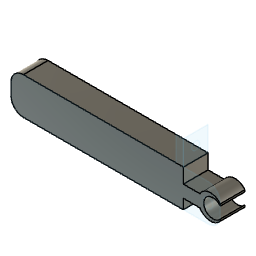
Current Final Hand Assembly (Autodesk Fusion 360 archive; units mm, degrees)
design "index_finger_new v3 (1) v2"
Autodesk Fusion 360 part; units mm, degrees
note: some values were not read from the file. Chosen so that the rebuilt part matches the saved one: where a step ends; which bodies a step acts on; which face or edge a step refers to. Set by a fixed rule: which sketch regions a step uses.
(part 1 of 5)
sketch "Sketch1" plane through (0, 0, 0) normal (0, 1, 0) x (1, 0, 0)
  line L0 (0, 0) -> (85, 0)
  line L1 (85, 0) -> (85, -15)
  line L2 (85, -15) -> (0, -15)
  line L3 (0, -15) -> (0, 0)
  dimension "d1" = 85
  dimension "d2" = 15
  constraint horizontal L0
  constraint vertical L1
  constraint horizontal L2
  constraint vertical L3
  constraint coincident L0.start L3.end
  measures "d1" distance of L0.start L0.end
  measures "d2" distance of L0.start L2.end
extrude "Extrude1" add sketch "Sketch1" along normal blind 10 makes body 1
fillet "Fillet1" radius 5 4 edges at (0, 5, 15) (0, 5, 0) (85, 5, 15) (85, 5, 0) on bodies 1
sketch "Sketch2" plane through (0, 0, 15) normal (0, 0, 1) x (-1, 0, 0)
  line L0 (-80, 0) -> (-80, -10)
  line L1 (-80, -10) -> (-5, -10)
  line L2 (-5, -10) -> (-5, 0)
  line L3 (-5, 0) -> (-80, 0)
  line L4 (-67, -10) -> (-70, -10)
  line L5 (-70, -10) -> (-70, 0)
  line L6 (-70, 0) -> (-67, 0)
  line L7 (-67, 0) -> (-67, -10)
  dimension "d7" = 3
  dimension "d8" = 10
  constraint horizontal L4
  constraint vertical L5
  constraint horizontal L6
  constraint vertical L7
  constraint coincident L1 L4.start
  measures "d7" distance of L4.start L4.end
  measures "d8" distance of L0 L5
extrude "Extrude2" add sketch "Sketch2" along normal blind 10 contours L1 L3 L4 L5 L6 L7 bodies 1
sketch "Sketch3" plane through (0, 0, 0) normal (0, -1, 0) x (1, 0, 0)
  arc A0 (80, 0) -> (85, 5) centre (80, 5) ccw
  line L0 (85, 5) -> (85, 10)
  arc A1 (85, 10) -> (80, 15) centre (80, 10) ccw
  line L1 (80, 15) -> (70, 15)
  line L2 (70, 15) -> (70, 25)
  line L3 (70, 25) -> (67, 25)
  line L4 (67, 25) -> (67, 15)
  line L5 (67, 15) -> (5, 15)
  arc A2 (5, 15) -> (0, 10) centre (5, 10) ccw
  line L6 (0, 10) -> (0, 5)
  arc A3 (0, 5) -> (5, 0) centre (5, 5) ccw
  line L7 (5, 0) -> (80, 0)
  circle A4 centre (80, 7.4726) radius 2
  dimension "d11" = 4
  measures "d11" diameter of A4
extrude "Extrude3" cut sketch "Sketch3" against normal blind 13 contours A4 bodies 1
sketch "Sketch4" plane through (70, 0, 0) normal (1, 0, 0) x (0, 1, 0)
  line L0 (0, 15) -> (10, 15)
  line L1 (10, 15) -> (10, 25)
  line L2 (10, 25) -> (0, 25)
  line L3 (0, 25) -> (0, 15)
  circle A0 centre (5, 20.0248) radius 1.625
  dimension "d14" = 3.25
  measures "d14" diameter of A0
extrude "Extrude4" cut sketch "Sketch4" against normal blind 56 contours A0 bodies 1
sketch "Sketch5" plane through (0, 0, 0) normal (0, -1, 0) x (1, 0, 0)
  circle A0 centre (80, 7.4726) radius 2
  arc A1 (80, 0) -> (85, 5) centre (80, 5) ccw
  line L0 (85, 5) -> (85, 10)
  arc A2 (85, 10) -> (80, 15) centre (80, 10) ccw
  line L1 (80, 15) -> (70, 15)
  line L2 (70, 15) -> (70, 25)
  line L3 (70, 25) -> (67, 25)
  line L4 (67, 25) -> (67, 15)
  line L5 (67, 15) -> (5, 15)
  arc A3 (5, 15) -> (0, 10) centre (5, 10) ccw
  line L6 (0, 10) -> (0, 5)
  arc A4 (0, 5) -> (5, 0) centre (5, 5) ccw
  line L7 (5, 0) -> (80, 0)
sketch "Sketch6" plane through (70, 0, 0) normal (1, 0, 0) x (0, 1, 0)
  circle A0 centre (5, 20.0248) radius 1.625
  line L0 (0, 15) -> (10, 15)
  line L1 (10, 15) -> (10, 25)
  line L2 (10, 25) -> (0, 25)
  line L3 (0, 25) -> (0, 15)
sketch "Sketch7" plane through (85, 0, 0) normal (1, 0, 0) x (0, 1, 0)
  line L0 (0, 5) -> (10, 5)
  line L1 (10, 5) -> (10, 10)
  line L2 (10, 10) -> (0, 10)
  line L3 (0, 10) -> (0, 5)
  line L4 (0, 15) -> (10, 15)
  line L5 (10, 15) -> (10, 0)
  line L6 (10, 0) -> (0, 0)
  line L7 (0, 0) -> (0, 15)
  constraint horizontal L4
  constraint vertical L5
  constraint horizontal L6
  constraint vertical L7
extrude "Extrude5" cut sketch "Sketch7" against normal blind 15 bodies 1
sketch "Sketch8" plane through (70, 0, 0) normal (1, 0, 0) x (0, 1, 0)
  circle A0 centre (5, 20.0248) radius 1.625
  line L0 (10, 0) -> (10, 25)
  line L1 (10, 25) -> (0, 25)
  line L2 (0, 25) -> (0, 0)
  line L3 (0, 0) -> (10, 0)
  line L4 (0, 9) -> (10, 9)
  line L5 (10, 9) -> (10, 4)
  line L6 (10, 4) -> (0, 4)
  line L7 (0, 4) -> (0, 9)
  line L8 (10, 25) -> (0, 25)
  dimension "d19" = 5
  dimension "d20" = 10
  dimension "d21" = 16
  constraint horizontal L4
  constraint vertical L5
  constraint horizontal L6
  constraint vertical L7
  constraint coincident L2 L4.start
  measures "d19" distance of L4.start L6.end
  measures "d20" distance of L4.start L4.end
  measures "d21" distance of L4 L8
extrude "Extrude6" add sketch "Sketch8" along normal blind 7.5 contours L0 L2 L4 L5 L6 L7 bodies 1
cylinder "CylinderPrimitive1" add diameter 10 height -10 placed x (1, 0, 0) y (0, 0, -1) z (0, 1, 0) at (81.0326, 10, 6.5) separate body makes body 2
ref_plane "WorkPlane1" through (87, 0, 0) normal (1, 0, 0) x (0, 1, 0)
sketch "Sketch11" plane through (87, 0, 0) normal (1, 0, 0) x (0, 1, 0)
  line L0 (-1.0999, 12.5133) -> (11, 12.5133)
  line L1 (11, 12.5133) -> (11, 1)
  line L2 (11, 1) -> (-1.0999, 1)
  line L3 (-1.0999, 1) -> (-1.0999, 12.5133)
  constraint horizontal L0
  constraint vertical L1
  constraint horizontal L2
  constraint vertical L3
extrude "Extrude7" cut sketch "Sketch11" against normal blind 2 bodies 2
copy_body "CopyPasteBodies1" bodies 2 makes body 3
move_body "Move1" bodies 3 to x (1, 0, 0) y (0, 1, 0) z (0, 0, 1) at (19, 0, 0)
scale "Scale1" factors (0.75, 1, 0.75) about (104, 0, 3.457) bodies 3
move_body "Move2" bodies 3 to x (1, 0, 0) y (0, 1, 0) z (0, 0, 1) at (-19, 0, 0.7608)
combine "Combine1" operation add target body 1 tool bodies 2
split "Split1" by bodies 3 bodies 1 makes body 4 at (47.3333, 10, 5)
move_body "Move3" bodies 1 to x (1, 0, 0) y (0, 1, 0) z (0, 0, 1) at (20, 0, 0)
sketch "Sketch12" plane through (0, 0, 0) normal (0, -1, 0) x (1, 0, 0)
sketch "Sketch15" plane through (67, 0, 0) normal (-1, 0, 0) x (0, -1, 0)
  circle A0 centre (-5, 20.0248) radius 1.625
  line L0 (-10, 15) -> (0, 15)
  line L1 (0, 15) -> (0, 25)
  line L2 (0, 25) -> (-10, 25)
  line L3 (-10, 25) -> (-10, 15)
  line L4 (-10, 25) -> (0, 25)
  line L5 (0, 25) -> (0, 15)
  line L6 (0, 15) -> (-10, 15)
  line L7 (-10, 15) -> (-10, 25)
  constraint horizontal L4
  constraint vertical L5
  constraint horizontal L6
  constraint vertical L7
  constraint coincident L0.end L1.start
  constraint coincident L2.end L3.start
extrude "Extrude8" cut sketch "Sketch15" against normal blind 10 bodies 4
sketch "Sketch19" plane through (0, 0, 0) normal (0, -1, 0) x (1, 0, 0)
hidden bodies 1 3

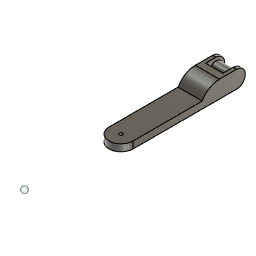
design "FingerOnly"
Autodesk Fusion 360 part; units mm, degrees
sketch "Sketch1" plane through (0, 0, 0) normal (0, 0, 1) x (1, 0, 0)
  circle A0 centre (0, 0) radius 7
  line L0 (-7, 0) -> (-7, 50.081)
  line L1 (-7, 50.081) -> (7, 50.081)
  line L2 (7, 50.081) -> (7, 0)
  dimension "d1" = 14
  dimension "d2" = 50.081
  dimension "d3" = 14
  dimension "d4" = 50.081
  constraint coincident A0.centre origin
  constraint coincident A0 L0.start
  constraint vertical L0
  constraint perpendicular L0 L1
  constraint coincident A0 L2.end
  constraint tangent A0 L2
  measures "d1" diameter of A0
  measures "d2" distance of L0.start L0.end
  measures "d3" distance of L0.end L1.end
  measures "d4" vertical distance of L1.end L2.end
extrude "Extrude1" add sketch "Sketch1" along normal blind 4
sketch "Sketch4" plane through (0, 0, 4) normal (0, 0, 1) x (-1, 0, 0)
  arc A0 (7, 0) -> (-7, 0) centre (0, 0) ccw
  line L0 (-7, 0) -> (-7, -50.081)
  line L1 (-7, -50.081) -> (7, -50.081)
  line L2 (7, -50.081) -> (7, 0)
  line L3 (-7, -50.081) -> (-7, -40.081)
  line L4 (7, -40.081) -> (7, -50.081)
  line L5 (-7, -40.081) -> (7, -40.081)
  dimension "d17" = 10
  constraint coincident L0.end L1.start
  constraint coincident L0 L3.end
  constraint perpendicular L1 L3
  constraint coincident L2 L4.start
  constraint coincident L1.end L2.start
  constraint perpendicular L1 L4
  constraint perpendicular L4 L5
  measures "d17" distance of L4.start L1.end
extrude "Extrude4" add sketch "Sketch4" along normal blind 6 contours L0 L1 L2 L3 L4 L5
fillet "Fillet1" radius 11.5 1 edges at (0, 40.081, 10)
sketch "Sketch5" plane through (-7, 0, 0) normal (-1, 0, 0) x (0, -1, 0)
  arc A0 (-40.081, 4) -> (-50.081, 10) centre (-50.1807, -1.4996) ccw
  line L0 (-50.081, 10) -> (-50.081, 0)
  line L1 (-50.081, 0) -> (0, 0)
  line L2 (0, 0) -> (0, 4)
  line L3 (0, 4) -> (-40.081, 4)
  line L4 (-50.081, 10) -> (-60.081, 10)
  line L5 (-60.081, 10) -> (-60.081, 0)
  line L6 (-60.081, 0) -> (-50.081, 0)
  dimension "d22" = 10
  constraint coincident A0.end L0.start
  constraint perpendicular L0 L4
  constraint perpendicular L4 L5
  constraint coincident L0.end L1.start
  constraint perpendicular L0 L6
  measures "d22" distance of A0.end L4.end
extrude "Extrude5" add sketch "Sketch5" against normal blind 2 contours L0 L4 L5 L6
sketch "Sketch6" plane through (7, 0, 0) normal (1, 0, 0) x (0, 1, 0)
  arc A0 (50.081, 10) -> (40.081, 4) centre (50.1807, -1.4996) ccw
  line L0 (40.081, 4) -> (0, 4)
  line L1 (0, 4) -> (0, 0)
  line L2 (0, 0) -> (50.081, 0)
  line L3 (50.081, 0) -> (50.081, 10)
  line L4 (50.081, 10) -> (60.081, 10)
  line L5 (60.081, 10) -> (60.081, 0)
  line L6 (60.081, 0) -> (50.081, 0)
  dimension "d25" = 10
  constraint coincident A0.start L3.end
  constraint perpendicular L3 L4
  constraint perpendicular L4 L5
  constraint coincident L2.end L3.start
  constraint perpendicular L3 L6
  measures "d25" distance of A0.start L4.end
extrude "Extrude6" add sketch "Sketch6" against normal blind 2 contours L3 L4 L5 L6
sketch "Sketch7" plane through (7, 0, 0) normal (1, 0, 0) x (0, 1, 0)
  arc A0 (50.081, 10) -> (40.081, 4) centre (50.1807, -1.4996) ccw
  line L0 (40.081, 4) -> (0, 4)
  line L1 (0, 4) -> (0, 0)
  line L2 (0, 0) -> (60.081, 0)
  line L3 (60.081, 0) -> (60.081, 10)
  line L4 (60.081, 10) -> (50.081, 10)
  circle A1 centre (60.081, 5) radius 5
  dimension "d28" = 10
  constraint midpoint L3 A1.centre
  measures "d28" diameter of A1
extrude "Extrude7" add sketch "Sketch7" against normal blind 2 contours L3 A1 picked at (62.1497, 5.5371)
sketch "Sketch8" plane through (-7, 0, 0) normal (-1, 0, 0) x (0, -1, 0)
  arc A0 (-40.081, 4) -> (-50.081, 10) centre (-50.1807, -1.4996) ccw
  line L0 (-50.081, 10) -> (-60.081, 10)
  line L1 (-60.081, 10) -> (-60.081, 0)
  line L2 (-60.081, 0) -> (0, 0)
  line L3 (0, 0) -> (0, 4)
  line L4 (0, 4) -> (-40.081, 4)
  circle A1 centre (-60.081, 5) radius 5
  dimension "d31" = 10
  constraint midpoint L1 A1.centre
  measures "d31" diameter of A1
extrude "Extrude8" add sketch "Sketch8" against normal blind 2 contours L1 A1 | L1 A1
extrude "Extrude9" add 1 faces at (1.6667, 50.081, 3.3332) along direction (0, 1, 0) blind 4
sketch "Sketch10" plane through (5, 0, 0) normal (-1, 0, 0) x (0, -1, 0)
  line L0 (-54.081, 0) -> (-54.081, 10)
  line L1 (-54.081, 10) -> (-60.081, 10)
  arc A0 (-60.081, 10) -> (-60.081, 0) centre (-60.081, 5) ccw
  line L2 (-60.081, 0) -> (-54.081, 0)
  circle A1 centre (-60.081, 5) radius 3.25
  dimension "d36" = 6.5
  constraint concentric A0 A1
  measures "d36" diameter of A1
extrude "Extrude10" add sketch "Sketch10" along normal up to far side of body 1 contours A1
move_body "Move1" bodies 1 to x (1, 0, 0) y (0, 1, 0) z (0, 0, 1) at (0, 28, 0)
sketch "Sketch12" plane through (0, 0, 4) normal (0, 0, -1) x (-1, 0, 0)
  circle A0 centre (0, -28) radius 1
  dimension "d43" = 2
  measures "d43" diameter of A0
sketch "Sketch13" plane through (0, 0, 4) normal (0, 0, 1) x (-1, 0, 0)
  line L0 (-7, -68.081) -> (7, -68.081)
  line L1 (7, -68.081) -> (7, -28)
  arc A0 (7, -28) -> (-7, -28) centre (0, -28) ccw
  line L2 (-7, -28) -> (-7, -68.081)
  circle A1 centre (0, -28) radius 1
  dimension "d44" = 2
  constraint concentric A0 A1
  measures "d44" diameter of A1
hole "Hole2" at (0, 28, 4) direction (0, 0, -1) diameter 2 depth 4 tip angle 118

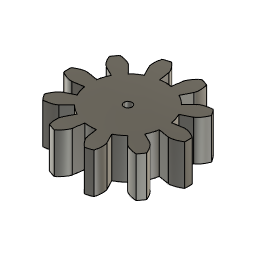
design "Gear10"
Autodesk Fusion 360 part; units mm, degrees
sketch "Sketch1" plane through (0, 0, 0) normal (0, 0, 1) x (1, 0, 0)
  spline S0 degree 5 poles (11.943507, -1.959599) (11.94367, -1.959624) (11.944019, -1.959676) (11.944609, -1.959763) (11.945532, -1.959893) (11.946908, -1.960081) (11.948507, -1.960293) (11.950325, -1.960527) (11.952355, -1.96078) (11.954593, -1.961049) (11.957034, -1.961331) (11.959673, -1.961624) (11.962506, -1.961927) (11.965532, -1.962238) (11.968746, -1.962554) (11.972145, -1.962875) (11.975726, -1.963198) (11.979485, -1.963522) (11.983419, -1.963845) (11.987526, -1.964165) (11.991802, -1.964481) (11.996245, -1.964792) (12.000852, -1.965096) (12.00562, -1.965392) (12.010548, -1.965678) (12.015633, -1.965954) (12.020871, -1.966218) (12.026262, -1.966468) (12.031803, -1.966704) (12.037491, -1.966925) (12.043325, -1.96713) (12.049302, -1.967316) (12.05542, -1.967485) (12.061679, -1.967633) (12.068075, -1.967761) (12.074606, -1.967868) (12.081272, -1.967952) (12.08807, -1.968014) (12.094999, -1.968051) (12.102057, -1.968063) (12.109241, -1.968049) (12.116552, -1.968009) (12.123986, -1.967941) (12.131544, -1.967845) (12.139222, -1.967721) (12.14702, -1.967567) (12.154935, -1.967382) (12.162968, -1.967167) (12.171116, -1.96692) (12.179378, -1.966641) (12.187753, -1.966329) (12.19624, -1.965983) (12.204836, -1.965603) (12.213541, -1.965189) (12.222354, -1.964739) (12.231273, -1.964253) (12.240298, -1.963731) (12.249427, -1.963171) (12.258658, -1.962575) (12.267992, -1.96194) (12.277426, -1.961266) (12.28696, -1.960554) (12.296592, -1.959801) (12.306322, -1.959009) (12.316148, -1.958176) (12.32607, -1.957303) (12.336086, -1.956387) (12.346195, -1.95543) (12.356398, -1.954431) (12.366691, -1.953389) (12.377075, -1.952304) (12.387549, -1.951175) (12.398111, -1.950002) (12.408762, -1.948785) (12.419499, -1.947523) (12.430322, -1.946216) (12.44123, -1.944863) (12.452223, -1.943465) (12.463299, -1.94202) (12.474458, -1.940529) (12.485698, -1.938991) (12.497019, -1.937405) (12.508421, -1.935772) (12.519902, -1.934091) (12.531461, -1.932362) (12.543099, -1.930585) (12.554813, -1.928758) (12.566604, -1.926883) (12.57847, -1.924957) (12.590411, -1.922983) (12.602426, -1.920958) (12.614514, -1.918883) (12.626675, -1.916757) (12.638908, -1.91458) (12.651212, -1.912353) (12.663586, -1.910074) (12.676031, -1.907743) (12.688544, -1.90536) (12.701127, -1.902925) (12.713776, -1.900438) (12.726493, -1.897899) (12.739277, -1.895306) (12.752126, -1.89266) (12.765041, -1.889961) (12.77802, -1.887209) (12.791064, -1.884402) (12.80417, -1.881542) (12.81734, -1.878627) (12.830571, -1.875659) (12.843864, -1.872635) (12.857218, -1.869557) (12.870632, -1.866424) (12.884106, -1.863235) (12.89764, -1.859991) (12.911232, -1.856692) (12.924882, -1.853337) (12.938589, -1.849925) (12.952353, -1.846458) (12.966174, -1.842935) (12.980051, -1.839355) (12.993982, -1.835718) (13.007969, -1.832025) (13.02201, -1.828274) (13.036104, -1.824467) (13.050251, -1.820602) (13.064451, -1.81668) (13.078704, -1.8127) (13.093007, -1.808662) (13.107362, -1.804567) (13.121768, -1.800413) (13.136223, -1.796202) (13.150728, -1.791932) (13.165282, -1.787603) (13.179884, -1.783216) (13.194535, -1.77877) (13.209233, -1.774266) (13.223979, -1.769702) (13.238771, -1.76508) (13.253609, -1.760398) (13.268493, -1.755657) (13.283422, -1.750856) (13.298395, -1.745996) (13.313413, -1.741076) (13.328475, -1.736096) (13.343581, -1.731056) (13.358729, -1.725956) (13.37392, -1.720797) (13.389152, -1.715577) (13.404427, -1.710296) (13.419742, -1.704955) (13.435098, -1.699554) (13.450495, -1.694092) (13.465931, -1.688569) (13.481407, -1.682985) (13.496921, -1.677341) (13.512475, -1.671635) (13.528066, -1.665869) (13.543695, -1.660041) (13.559362, -1.654152) (13.575065, -1.648201) (13.590805, -1.64219) (13.606581, -1.636116) (13.622393, -1.629981) (13.63824, -1.623785) (13.654122, -1.617526) (13.670038, -1.611206) (13.685988, -1.604824) (13.701972, -1.59838) (13.71799, -1.591874) (13.73404, -1.585306) (13.750123, -1.578676) (13.766238, -1.571984) (13.782385, -1.565229) (13.798563, -1.558412) (13.814772, -1.551532) (13.831012, -1.54459) (13.847282, -1.537586) (13.863582, -1.530519) (13.879911, -1.523389) (13.89627, -1.516197) (13.912657, -1.508942) (13.929073, -1.501624) (13.945517, -1.494244) (13.961988, -1.4868) (13.978487, -1.479294) (13.995013, -1.471724) (14.011565, -1.464092) (14.028144, -1.456396) (14.044749, -1.448638) (14.061379, -1.440816) (14.078034, -1.432931) (14.094714, -1.424983) (14.111419, -1.416972) (14.128148, -1.408897) (14.144901, -1.400759) (14.161678, -1.392558) (14.178477, -1.384293) (14.1953, -1.375965) (14.212145, -1.367574) (14.229012, -1.359119) (14.245901, -1.3506) (14.262812, -1.342018) (14.279743, -1.333373) (14.296696, -1.324663) (14.313669, -1.315891) (14.330662, -1.307054) (14.347676, -1.298154) (14.364708, -1.28919) (14.381761, -1.280163) (14.398832, -1.271072) (14.415921, -1.261917) (14.433029, -1.252698) (14.450155, -1.243416) (14.467299, -1.234069) (14.48446, -1.22466) (14.501638, -1.215186) (14.518833, -1.205648) (14.536045, -1.196047) (14.553272, -1.186381) (14.570516, -1.176652) (14.587775, -1.166859) (14.605049, -1.157003) (14.622338, -1.147082) (14.639642, -1.137097) (14.65696, -1.127049) (14.674292, -1.116936) (14.691638, -1.10676) (14.708998, -1.09652) (14.72637, -1.086216) (14.743756, -1.075848) (14.761155, -1.065416) (14.778565, -1.054921) (14.795988, -1.044361) (14.813423, -1.033738) (14.830868, -1.02305) (14.848325, -1.012299) (14.865793, -1.001484) (14.883271, -0.990605) (14.900759, -0.979662) (14.918257, -0.968655) (14.935766, -0.957584) (14.949781, -0.948677) (14.960297, -0.941967) (14.967309, -0.937482) (14.970816, -0.935235) knots 0 0 0 0 0 0 0.00416667 0.00833333 0.0125 0.01666667 0.02083333 0.025 0.02916667 0.03333333 0.0375 0.04166667 0.04583333 0.05 0.05416667 0.05833333 0.0625 0.06666667 0.07083333 0.075 0.07916667 0.08333333 0.0875 0.09166667 0.09583333 0.1 0.10416667 0.10833333 0.1125 0.11666667 0.12083333 0.125 0.12916667 0.13333333 0.1375 0.14166667 0.14583333 0.15 0.15416667 0.15833333 0.1625 0.16666667 0.17083333 0.175 0.17916667 0.18333333 0.1875 0.19166667 0.19583333 0.2 0.20416667 0.20833333 0.2125 0.21666667 0.22083333 0.225 0.22916667 0.23333333 0.2375 0.24166667 0.24583333 0.25 0.25416667 0.25833333 0.2625 0.26666667 0.27083333 0.275 0.27916667 0.28333333 0.2875 0.29166667 0.29583333 0.3 0.30416667 0.30833333 0.3125 0.31666667 0.32083333 0.325 0.32916667 0.33333333 0.3375 0.34166667 0.34583333 0.35 0.35416667 0.35833333 0.3625 0.36666667 0.37083333 0.375 0.37916667 0.38333333 0.3875 0.39166667 0.39583333 0.4 0.40416667 0.40833333 0.4125 0.41666667 0.42083333 0.425 0.42916667 0.43333333 0.4375 0.44166667 0.44583333 0.45 0.45416667 0.45833333 0.4625 0.46666667 0.47083333 0.475 0.47916667 0.48333333 0.4875 0.49166667 0.49583333 0.5 0.50416667 0.50833333 0.5125 0.51666667 0.52083333 0.525 0.52916667 0.53333333 0.5375 0.54166667 0.54583333 0.55 0.55416667 0.55833333 0.5625 0.56666667 0.57083333 0.575 0.57916667 0.58333333 0.5875 0.59166667 0.59583333 0.6 0.60416667 0.60833333 0.6125 0.61666667 0.62083333 0.625 0.62916667 0.63333333 0.6375 0.64166667 0.64583333 0.65 0.65416667 0.65833333 0.6625 0.66666667 0.67083333 0.675 0.67916667 0.68333333 0.6875 0.69166667 0.69583333 0.7 0.70416667 0.70833333 0.7125 0.71666667 0.72083333 0.725 0.72916667 0.73333333 0.7375 0.74166667 0.74583333 0.75 0.75416667 0.75833333 0.7625 0.76666667 0.77083333 0.775 0.77916667 0.78333333 0.7875 0.79166667 0.79583333 0.8 0.80416667 0.80833333 0.8125 0.81666667 0.82083333 0.825 0.82916667 0.83333333 0.8375 0.84166667 0.84583333 0.85 0.85416667 0.85833333 0.8625 0.86666667 0.87083333 0.875 0.87916667 0.88333333 0.8875 0.89166667 0.89583333 0.9 0.90416667 0.90833333 0.9125 0.91666667 0.92083333 0.925 0.92916667 0.93333333 0.9375 0.94166667 0.94583333 0.95 0.95416667 0.95833333 0.9625 0.96666667 0.97083333 0.975 0.97916667 0.98333333 0.9875 0.99166667 0.99583333 1 1 1 1 1 1
  spline S1 degree 5 poles (11.943507, 1.959599) (11.94367, 1.959624) (11.944019, 1.959676) (11.944609, 1.959763) (11.945532, 1.959893) (11.946908, 1.960081) (11.948507, 1.960293) (11.950325, 1.960527) (11.952355, 1.96078) (11.954593, 1.961049) (11.957034, 1.961331) (11.959673, 1.961624) (11.962506, 1.961927) (11.965532, 1.962238) (11.968746, 1.962554) (11.972145, 1.962875) (11.975726, 1.963198) (11.979485, 1.963522) (11.983419, 1.963845) (11.987526, 1.964165) (11.991802, 1.964481) (11.996245, 1.964792) (12.000852, 1.965096) (12.00562, 1.965392) (12.010548, 1.965678) (12.015633, 1.965954) (12.020871, 1.966218) (12.026262, 1.966468) (12.031803, 1.966704) (12.037491, 1.966925) (12.043325, 1.96713) (12.049302, 1.967316) (12.05542, 1.967485) (12.061679, 1.967633) (12.068075, 1.967761) (12.074606, 1.967868) (12.081272, 1.967952) (12.08807, 1.968014) (12.094999, 1.968051) (12.102057, 1.968063) (12.109241, 1.968049) (12.116552, 1.968009) (12.123986, 1.967941) (12.131544, 1.967845) (12.139222, 1.967721) (12.14702, 1.967567) (12.154935, 1.967382) (12.162968, 1.967167) (12.171116, 1.96692) (12.179378, 1.966641) (12.187753, 1.966329) (12.19624, 1.965983) (12.204836, 1.965603) (12.213541, 1.965189) (12.222354, 1.964739) (12.231273, 1.964253) (12.240298, 1.963731) (12.249427, 1.963171) (12.258658, 1.962575) (12.267992, 1.96194) (12.277426, 1.961266) (12.28696, 1.960554) (12.296592, 1.959801) (12.306322, 1.959009) (12.316148, 1.958176) (12.32607, 1.957303) (12.336086, 1.956387) (12.346195, 1.95543) (12.356398, 1.954431) (12.366691, 1.953389) (12.377075, 1.952304) (12.387549, 1.951175) (12.398111, 1.950002) (12.408762, 1.948785) (12.419499, 1.947523) (12.430322, 1.946216) (12.44123, 1.944863) (12.452223, 1.943465) (12.463299, 1.94202) (12.474458, 1.940529) (12.485698, 1.938991) (12.497019, 1.937405) (12.508421, 1.935772) (12.519902, 1.934091) (12.531461, 1.932362) (12.543099, 1.930585) (12.554813, 1.928758) (12.566604, 1.926883) (12.57847, 1.924957) (12.590411, 1.922983) (12.602426, 1.920958) (12.614514, 1.918883) (12.626675, 1.916757) (12.638908, 1.91458) (12.651212, 1.912353) (12.663586, 1.910074) (12.676031, 1.907743) (12.688544, 1.90536) (12.701127, 1.902925) (12.713776, 1.900438) (12.726493, 1.897899) (12.739277, 1.895306) (12.752126, 1.89266) (12.765041, 1.889961) (12.77802, 1.887209) (12.791064, 1.884402) (12.80417, 1.881542) (12.81734, 1.878627) (12.830571, 1.875659) (12.843864, 1.872635) (12.857218, 1.869557) (12.870632, 1.866424) (12.884106, 1.863235) (12.89764, 1.859991) (12.911232, 1.856692) (12.924882, 1.853337) (12.938589, 1.849925) (12.952353, 1.846458) (12.966174, 1.842935) (12.980051, 1.839355) (12.993982, 1.835718) (13.007969, 1.832025) (13.02201, 1.828274) (13.036104, 1.824467) (13.050251, 1.820602) (13.064451, 1.81668) (13.078704, 1.8127) (13.093007, 1.808662) (13.107362, 1.804567) (13.121768, 1.800413) (13.136223, 1.796202) (13.150728, 1.791932) (13.165282, 1.787603) (13.179884, 1.783216) (13.194535, 1.77877) (13.209233, 1.774266) (13.223979, 1.769702) (13.238771, 1.76508) (13.253609, 1.760398) (13.268493, 1.755657) (13.283422, 1.750856) (13.298395, 1.745996) (13.313413, 1.741076) (13.328475, 1.736096) (13.343581, 1.731056) (13.358729, 1.725956) (13.37392, 1.720797) (13.389152, 1.715577) (13.404427, 1.710296) (13.419742, 1.704955) (13.435098, 1.699554) (13.450495, 1.694092) (13.465931, 1.688569) (13.481407, 1.682985) (13.496921, 1.677341) (13.512475, 1.671635) (13.528066, 1.665869) (13.543695, 1.660041) (13.559362, 1.654152) (13.575065, 1.648201) (13.590805, 1.64219) (13.606581, 1.636116) (13.622393, 1.629981) (13.63824, 1.623785) (13.654122, 1.617526) (13.670038, 1.611206) (13.685988, 1.604824) (13.701972, 1.59838) (13.71799, 1.591874) (13.73404, 1.585306) (13.750123, 1.578676) (13.766238, 1.571984) (13.782385, 1.565229) (13.798563, 1.558412) (13.814772, 1.551532) (13.831012, 1.54459) (13.847282, 1.537586) (13.863582, 1.530519) (13.879911, 1.523389) (13.89627, 1.516197) (13.912657, 1.508942) (13.929073, 1.501624) (13.945517, 1.494244) (13.961988, 1.4868) (13.978487, 1.479294) (13.995013, 1.471724) (14.011565, 1.464092) (14.028144, 1.456396) (14.044749, 1.448638) (14.061379, 1.440816) (14.078034, 1.432931) (14.094714, 1.424983) (14.111419, 1.416972) (14.128148, 1.408897) (14.144901, 1.400759) (14.161678, 1.392558) (14.178477, 1.384293) (14.1953, 1.375965) (14.212145, 1.367574) (14.229012, 1.359119) (14.245901, 1.3506) (14.262812, 1.342018) (14.279743, 1.333373) (14.296696, 1.324663) (14.313669, 1.315891) (14.330662, 1.307054) (14.347676, 1.298154) (14.364708, 1.28919) (14.381761, 1.280163) (14.398832, 1.271072) (14.415921, 1.261917) (14.433029, 1.252698) (14.450155, 1.243416) (14.467299, 1.234069) (14.48446, 1.22466) (14.501638, 1.215186) (14.518833, 1.205648) (14.536045, 1.196047) (14.553272, 1.186381) (14.570516, 1.176652) (14.587775, 1.166859) (14.605049, 1.157003) (14.622338, 1.147082) (14.639642, 1.137097) (14.65696, 1.127049) (14.674292, 1.116936) (14.691638, 1.10676) (14.708998, 1.09652) (14.72637, 1.086216) (14.743756, 1.075848) (14.761155, 1.065416) (14.778565, 1.054921) (14.795988, 1.044361) (14.813423, 1.033738) (14.830868, 1.02305) (14.848325, 1.012299) (14.865793, 1.001484) (14.883271, 0.990605) (14.900759, 0.979662) (14.918257, 0.968655) (14.935766, 0.957584) (14.949781, 0.948677) (14.960297, 0.941967) (14.967309, 0.937482) (14.970816, 0.935235) knots 0 0 0 0 0 0 0.00416667 0.00833333 0.0125 0.01666667 0.02083333 0.025 0.02916667 0.03333333 0.0375 0.04166667 0.04583333 0.05 0.05416667 0.05833333 0.0625 0.06666667 0.07083333 0.075 0.07916667 0.08333333 0.0875 0.09166667 0.09583333 0.1 0.10416667 0.10833333 0.1125 0.11666667 0.12083333 0.125 0.12916667 0.13333333 0.1375 0.14166667 0.14583333 0.15 0.15416667 0.15833333 0.1625 0.16666667 0.17083333 0.175 0.17916667 0.18333333 0.1875 0.19166667 0.19583333 0.2 0.20416667 0.20833333 0.2125 0.21666667 0.22083333 0.225 0.22916667 0.23333333 0.2375 0.24166667 0.24583333 0.25 0.25416667 0.25833333 0.2625 0.26666667 0.27083333 0.275 0.27916667 0.28333333 0.2875 0.29166667 0.29583333 0.3 0.30416667 0.30833333 0.3125 0.31666667 0.32083333 0.325 0.32916667 0.33333333 0.3375 0.34166667 0.34583333 0.35 0.35416667 0.35833333 0.3625 0.36666667 0.37083333 0.375 0.37916667 0.38333333 0.3875 0.39166667 0.39583333 0.4 0.40416667 0.40833333 0.4125 0.41666667 0.42083333 0.425 0.42916667 0.43333333 0.4375 0.44166667 0.44583333 0.45 0.45416667 0.45833333 0.4625 0.46666667 0.47083333 0.475 0.47916667 0.48333333 0.4875 0.49166667 0.49583333 0.5 0.50416667 0.50833333 0.5125 0.51666667 0.52083333 0.525 0.52916667 0.53333333 0.5375 0.54166667 0.54583333 0.55 0.55416667 0.55833333 0.5625 0.56666667 0.57083333 0.575 0.57916667 0.58333333 0.5875 0.59166667 0.59583333 0.6 0.60416667 0.60833333 0.6125 0.61666667 0.62083333 0.625 0.62916667 0.63333333 0.6375 0.64166667 0.64583333 0.65 0.65416667 0.65833333 0.6625 0.66666667 0.67083333 0.675 0.67916667 0.68333333 0.6875 0.69166667 0.69583333 0.7 0.70416667 0.70833333 0.7125 0.71666667 0.72083333 0.725 0.72916667 0.73333333 0.7375 0.74166667 0.74583333 0.75 0.75416667 0.75833333 0.7625 0.76666667 0.77083333 0.775 0.77916667 0.78333333 0.7875 0.79166667 0.79583333 0.8 0.80416667 0.80833333 0.8125 0.81666667 0.82083333 0.825 0.82916667 0.83333333 0.8375 0.84166667 0.84583333 0.85 0.85416667 0.85833333 0.8625 0.86666667 0.87083333 0.875 0.87916667 0.88333333 0.8875 0.89166667 0.89583333 0.9 0.90416667 0.90833333 0.9125 0.91666667 0.92083333 0.925 0.92916667 0.93333333 0.9375 0.94166667 0.94583333 0.95 0.95416667 0.95833333 0.9625 0.96666667 0.97083333 0.975 0.97916667 0.98333333 0.9875 0.99166667 0.99583333 1 1 1 1 1 1
  spline S2 degree 5 poles (11.942171, -1.959393) (11.942224, -1.959401) (11.942331, -1.959418) (11.942491, -1.959442) (11.942705, -1.959475) (11.942972, -1.959516) (11.943186, -1.959549) (11.943346, -1.959574) (11.943453, -1.95959) (11.943507, -1.959599) knots 0 0 0 0 0 0 0.2 0.4 0.6 0.8 1 1 1 1 1 1
  spline S3 degree 5 poles (11.942171, 1.959393) (11.942224, 1.959401) (11.942331, 1.959418) (11.942491, 1.959442) (11.942705, 1.959475) (11.942972, 1.959516) (11.943186, 1.959549) (11.943346, 1.959574) (11.943453, 1.95959) (11.943507, 1.959599) knots 0 0 0 0 0 0 0.2 0.4 0.6 0.8 1 1 1 1 1 1
  line L0 (0, 0) -> (11.942171, -1.959393)
  line L1 (0, 0) -> (11.942171, 1.959393)
  arc A0 (14.970816, -0.935235) -> (14.970816, 0.935235) centre (0, 0) ccw
  point P0 (11.947522, -1.960162)
  point P1 (11.954228, -1.961003)
  point P2 (11.963631, -1.962041)
  point P3 (11.975741, -1.963196)
  point P4 (11.99056, -1.964387)
  point P5 (12.008093, -1.965533)
  point P6 (12.028342, -1.966554)
  point P7 (12.051304, -1.967368)
  point P8 (12.076979, -1.967895)
  point P9 (12.105361, -1.968053)
  point P10 (12.136447, -1.967762)
  point P11 (12.170226, -1.966941)
  point P12 (12.206691, -1.96551)
  point P13 (12.245829, -1.963388)
  point P14 (12.287628, -1.960494)
  point P15 (12.332073, -1.95675)
  point P16 (12.379147, -1.952074)
  point P17 (12.428831, -1.946389)
  point P18 (12.481106, -1.939614)
  point P19 (12.535948, -1.931672)
  point P20 (12.593336, -1.922484)
  point P21 (12.653241, -1.911972)
  point P22 (12.715639, -1.900059)
  point P23 (12.780499, -1.886668)
  point P24 (12.84779, -1.871724)
  point P25 (12.91748, -1.855151)
  point P26 (12.989535, -1.836873)
  point P27 (13.063919, -1.816817)
  point P28 (13.140594, -1.794909)
  point P29 (13.21952, -1.771076)
  point P30 (13.300658, -1.745246)
  point P31 (13.383964, -1.717348)
  point P32 (13.469393, -1.687312)
  point P33 (13.556901, -1.655068)
  point P34 (13.646439, -1.620548)
  point P35 (13.737959, -1.583683)
  point P36 (13.83141, -1.544407)
  point P37 (13.926739, -1.502655)
  point P38 (14.023894, -1.458361)
  point P39 (14.122818, -1.411463)
  point P40 (14.223455, -1.361897)
  point P41 (14.325747, -1.309602)
  point P42 (14.429635, -1.254518)
  point P43 (14.535057, -1.196586)
  point P44 (14.64195, -1.135747)
  point P45 (14.750252, -1.071946)
  point P46 (14.859896, -1.005127)
  point P47 (11.947522, 1.960162)
  point P48 (11.954228, 1.961003)
  point P49 (11.963631, 1.962041)
  point P50 (11.975741, 1.963196)
  point P51 (11.99056, 1.964387)
  point P52 (12.008093, 1.965533)
  point P53 (12.028342, 1.966554)
  point P54 (12.051304, 1.967368)
  point P55 (12.076979, 1.967895)
  point P56 (12.105361, 1.968053)
  point P57 (12.136447, 1.967762)
  point P58 (12.170226, 1.966941)
  point P59 (12.206691, 1.96551)
  point P60 (12.245829, 1.963388)
  point P61 (12.287628, 1.960494)
  point P62 (12.332073, 1.95675)
  point P63 (12.379147, 1.952074)
  point P64 (12.428831, 1.946389)
  point P65 (12.481106, 1.939614)
  point P66 (12.535948, 1.931672)
  point P67 (12.593336, 1.922484)
  point P68 (12.653241, 1.911972)
  point P69 (12.715639, 1.900059)
  point P70 (12.780499, 1.886668)
  point P71 (12.84779, 1.871724)
  point P72 (12.91748, 1.855151)
  point P73 (12.989535, 1.836873)
  point P74 (13.063919, 1.816817)
  point P75 (13.140594, 1.794909)
  point P76 (13.21952, 1.771076)
  point P77 (13.300658, 1.745246)
  point P78 (13.383964, 1.717348)
  point P79 (13.469393, 1.687312)
  point P80 (13.556901, 1.655068)
  point P81 (13.646439, 1.620548)
  point P82 (13.737959, 1.583683)
  point P83 (13.83141, 1.544407)
  point P84 (13.926739, 1.502655)
  point P85 (14.023894, 1.458361)
  point P86 (14.122818, 1.411463)
  point P87 (14.223455, 1.361897)
  point P88 (14.325747, 1.309602)
  point P89 (14.429635, 1.254518)
  point P90 (14.535057, 1.196586)
  point P91 (14.64195, 1.135747)
  point P92 (14.750252, 1.071946)
  point P93 (14.859896, 1.005127)
sketch "Sketch2" plane through (0, 0, 0) normal (0, 0, 1) x (1, 0, 0)
  circle A0 centre (0, 0) radius 9.375
extrude "Extrude1" add sketch "Sketch2" along normal blind 10 makes body 1
extrude "Extrude2" add sketch "Sketch1" along normal blind 10 separate body makes body 2
pattern_circular "C-Pattern1" count 10 over 360 about axis through (0, 0, 1.75) along (0, 0, 1) of "Extrude2" makes body 3 makes body 4 makes body 5 makes body 6 makes body 7 makes body 8 makes body 9 makes body 10 makes body 11
combine "Combine1" operation add target body 1 tool bodies 2 3 4 5 6 7 8 9 10 11
sketch "Sketch3" plane through (0, 0, 0) normal (0, 0, 1) x (1, 0, 0)
  line L0 (0, 0) -> (48.300295, 0) construction
  line L1 (48.300295, 0) -> (48.300295, 3) construction
  line L2 (48.300295, 3) -> (0, 3) construction
  line L3 (0, 3) -> (0, 0) construction
  constraint perpendicular L0 L1
  constraint parallel L0 L2
  constraint parallel L1 L3
sketch "Sketch4" plane through (0, 0, 10) normal (0, 0, 1) x (-1, 0, 0)
  arc A0 (-8.376657, 4.209779) -> (-9.251304, 1.517893) centre (0, 0) ccw
  line L0 (-9.251304, 1.517893) -> (-11.942171, 1.959393)
  line L1 (-11.942171, 1.959393) -> (-11.943507, 1.959599)
  spline S0 degree 5 poles (-11.943507, 1.959599) (-11.94367, 1.959624) (-11.944019, 1.959676) (-11.944609, 1.959763) (-11.945532, 1.959893) (-11.946908, 1.960081) (-11.948507, 1.960293) (-11.950325, 1.960527) (-11.952355, 1.96078) (-11.954593, 1.961049) (-11.957034, 1.961331) (-11.959673, 1.961624) (-11.962506, 1.961927) (-11.965532, 1.962238) (-11.968746, 1.962554) (-11.972145, 1.962875) (-11.975726, 1.963198) (-11.979485, 1.963522) (-11.983419, 1.963845) (-11.987526, 1.964165) (-11.991802, 1.964481) (-11.996245, 1.964792) (-12.000852, 1.965096) (-12.00562, 1.965392) (-12.010548, 1.965678) (-12.015633, 1.965954) (-12.020871, 1.966218) (-12.026262, 1.966468) (-12.031803, 1.966704) (-12.037491, 1.966925) (-12.043325, 1.96713) (-12.049302, 1.967316) (-12.05542, 1.967485) (-12.061679, 1.967633) (-12.068075, 1.967761) (-12.074606, 1.967868) (-12.081272, 1.967952) (-12.08807, 1.968014) (-12.094999, 1.968051) (-12.102057, 1.968063) (-12.109241, 1.968049) (-12.116552, 1.968009) (-12.123986, 1.967941) (-12.131544, 1.967845) (-12.139222, 1.967721) (-12.14702, 1.967567) (-12.154935, 1.967382) (-12.162968, 1.967167) (-12.171116, 1.96692) (-12.179378, 1.966641) (-12.187753, 1.966329) (-12.19624, 1.965983) (-12.204836, 1.965603) (-12.213541, 1.965189) (-12.222354, 1.964739) (-12.231273, 1.964253) (-12.240298, 1.963731) (-12.249427, 1.963171) (-12.258658, 1.962575) (-12.267992, 1.96194) (-12.277426, 1.961266) (-12.28696, 1.960554) (-12.296592, 1.959801) (-12.306322, 1.959009) (-12.316148, 1.958176) (-12.32607, 1.957303) (-12.336086, 1.956387) (-12.346195, 1.95543) (-12.356398, 1.954431) (-12.366691, 1.953389) (-12.377075, 1.952304) (-12.387549, 1.951175) (-12.398111, 1.950002) (-12.408762, 1.948785) (-12.419499, 1.947523) (-12.430322, 1.946216) (-12.44123, 1.944863) (-12.452223, 1.943465) (-12.463299, 1.94202) (-12.474458, 1.940529) (-12.485698, 1.938991) (-12.497019, 1.937405) (-12.508421, 1.935772) (-12.519902, 1.934091) (-12.531461, 1.932362) (-12.543099, 1.930585) (-12.554813, 1.928758) (-12.566604, 1.926883) (-12.57847, 1.924957) (-12.590411, 1.922983) (-12.602426, 1.920958) (-12.614514, 1.918883) (-12.626675, 1.916757) (-12.638908, 1.91458) (-12.651212, 1.912353) (-12.663586, 1.910074) (-12.676031, 1.907743) (-12.688544, 1.90536) (-12.701127, 1.902925) (-12.713776, 1.900438) (-12.726493, 1.897899) (-12.739277, 1.895306) (-12.752126, 1.89266) (-12.765041, 1.889961) (-12.77802, 1.887209) (-12.791064, 1.884402) (-12.80417, 1.881542) (-12.81734, 1.878627) (-12.830571, 1.875659) (-12.843864, 1.872635) (-12.857218, 1.869557) (-12.870632, 1.866424) (-12.884106, 1.863235) (-12.89764, 1.859991) (-12.911232, 1.856692) (-12.924882, 1.853337) (-12.938589, 1.849925) (-12.952353, 1.846458) (-12.966174, 1.842935) (-12.980051, 1.839355) (-12.993982, 1.835718) (-13.007969, 1.832025) (-13.02201, 1.828274) (-13.036104, 1.824467) (-13.050251, 1.820602) (-13.064451, 1.81668) (-13.078704, 1.8127) (-13.093007, 1.808662) (-13.107362, 1.804567) (-13.121768, 1.800413) (-13.136223, 1.796202) (-13.150728, 1.791932) (-13.165282, 1.787603) (-13.179884, 1.783216) (-13.194535, 1.77877) (-13.209233, 1.774266) (-13.223979, 1.769702) (-13.238771, 1.76508) (-13.253609, 1.760398) (-13.268493, 1.755657) (-13.283422, 1.750856) (-13.298395, 1.745996) (-13.313413, 1.741076) (-13.328475, 1.736096) (-13.343581, 1.731056) (-13.358729, 1.725956) (-13.37392, 1.720797) (-13.389152, 1.715577) (-13.404427, 1.710296) (-13.419742, 1.704955) (-13.435098, 1.699554) (-13.450495, 1.694092) (-13.465931, 1.688569) (-13.481407, 1.682985) (-13.496921, 1.677341) (-13.512475, 1.671635) (-13.528066, 1.665869) (-13.543695, 1.660041) (-13.559362, 1.654152) (-13.575065, 1.648201) (-13.590805, 1.64219) (-13.606581, 1.636116) (-13.622393, 1.629981) (-13.63824, 1.623785) (-13.654122, 1.617526) (-13.670038, 1.611206) (-13.685988, 1.604824) (-13.701972, 1.59838) (-13.71799, 1.591874) (-13.73404, 1.585306) (-13.750123, 1.578676) (-13.766238, 1.571984) (-13.782385, 1.565229) (-13.798563, 1.558412) (-13.814772, 1.551532) (-13.831012, 1.54459) (-13.847282, 1.537586) (-13.863582, 1.530519) (-13.879911, 1.523389) (-13.89627, 1.516197) (-13.912657, 1.508942) (-13.929073, 1.501624) (-13.945517, 1.494244) (-13.961988, 1.4868) (-13.978487, 1.479294) (-13.995013, 1.471724) (-14.011565, 1.464092) (-14.028144, 1.456396) (-14.044749, 1.448638) (-14.061379, 1.440816) (-14.078034, 1.432931) (-14.094714, 1.424983) (-14.111419, 1.416972) (-14.128148, 1.408897) (-14.144901, 1.400759) (-14.161678, 1.392558) (-14.178477, 1.384293) (-14.1953, 1.375965) (-14.212145, 1.367574) (-14.229012, 1.359119) (-14.245901, 1.3506) (-14.262812, 1.342018) (-14.279743, 1.333373) (-14.296696, 1.324663) (-14.313669, 1.315891) (-14.330662, 1.307054) (-14.347676, 1.298154) (-14.364708, 1.28919) (-14.381761, 1.280163) (-14.398832, 1.271072) (-14.415921, 1.261917) (-14.433029, 1.252698) (-14.450155, 1.243416) (-14.467299, 1.234069) (-14.48446, 1.22466) (-14.501638, 1.215186) (-14.518833, 1.205648) (-14.536045, 1.196047) (-14.553272, 1.186381) (-14.570516, 1.176652) (-14.587775, 1.166859) (-14.605049, 1.157003) (-14.622338, 1.147082) (-14.639642, 1.137097) (-14.65696, 1.127049) (-14.674292, 1.116936) (-14.691638, 1.10676) (-14.708998, 1.09652) (-14.72637, 1.086216) (-14.743756, 1.075848) (-14.761155, 1.065416) (-14.778565, 1.054921) (-14.795988, 1.044361) (-14.813423, 1.033738) (-14.830868, 1.02305) (-14.848325, 1.012299) (-14.865793, 1.001484) (-14.883271, 0.990605) (-14.900759, 0.979662) (-14.918257, 0.968655) (-14.935766, 0.957584) (-14.949781, 0.948677) (-14.960297, 0.941967) (-14.967309, 0.937482) (-14.970816, 0.935235) knots 0 0 0 0 0 0 0.00416667 0.00833333 0.0125 0.01666667 0.02083333 0.025 0.02916667 0.03333333 0.0375 0.04166667 0.04583333 0.05 0.05416667 0.05833333 0.0625 0.06666667 0.07083333 0.075 0.07916667 0.08333333 0.0875 0.09166667 0.09583333 0.1 0.10416667 0.10833333 0.1125 0.11666667 0.12083333 0.125 0.12916667 0.13333333 0.1375 0.14166667 0.14583333 0.15 0.15416667 0.15833333 0.1625 0.16666667 0.17083333 0.175 0.17916667 0.18333333 0.1875 0.19166667 0.19583333 0.2 0.20416667 0.20833333 0.2125 0.21666667 0.22083333 0.225 0.22916667 0.23333333 0.2375 0.24166667 0.24583333 0.25 0.25416667 0.25833333 0.2625 0.26666667 0.27083333 0.275 0.27916667 0.28333333 0.2875 0.29166667 0.29583333 0.3 0.30416667 0.30833333 0.3125 0.31666667 0.32083333 0.325 0.32916667 0.33333333 0.3375 0.34166667 0.34583333 0.35 0.35416667 0.35833333 0.3625 0.36666667 0.37083333 0.375 0.37916667 0.38333333 0.3875 0.39166667 0.39583333 0.4 0.40416667 0.40833333 0.4125 0.41666667 0.42083333 0.425 0.42916667 0.43333333 0.4375 0.44166667 0.44583333 0.45 0.45416667 0.45833333 0.4625 0.46666667 0.47083333 0.475 0.47916667 0.48333333 0.4875 0.49166667 0.49583333 0.5 0.50416667 0.50833333 0.5125 0.51666667 0.52083333 0.525 0.52916667 0.53333333 0.5375 0.54166667 0.54583333 0.55 0.55416667 0.55833333 0.5625 0.56666667 0.57083333 0.575 0.57916667 0.58333333 0.5875 0.59166667 0.59583333 0.6 0.60416667 0.60833333 0.6125 0.61666667 0.62083333 0.625 0.62916667 0.63333333 0.6375 0.64166667 0.64583333 0.65 0.65416667 0.65833333 0.6625 0.66666667 0.67083333 0.675 0.67916667 0.68333333 0.6875 0.69166667 0.69583333 0.7 0.70416667 0.70833333 0.7125 0.71666667 0.72083333 0.725 0.72916667 0.73333333 0.7375 0.74166667 0.74583333 0.75 0.75416667 0.75833333 0.7625 0.76666667 0.77083333 0.775 0.77916667 0.78333333 0.7875 0.79166667 0.79583333 0.8 0.80416667 0.80833333 0.8125 0.81666667 0.82083333 0.825 0.82916667 0.83333333 0.8375 0.84166667 0.84583333 0.85 0.85416667 0.85833333 0.8625 0.86666667 0.87083333 0.875 0.87916667 0.88333333 0.8875 0.89166667 0.89583333 0.9 0.90416667 0.90833333 0.9125 0.91666667 0.92083333 0.925 0.92916667 0.93333333 0.9375 0.94166667 0.94583333 0.95 0.95416667 0.95833333 0.9625 0.96666667 0.97083333 0.975 0.97916667 0.98333333 0.9875 0.99166667 0.99583333 1 1 1 1 1 1
  arc A1 (-14.970816, 0.935235) -> (-14.970816, -0.935235) centre (0, 0) ccw
  spline S1 degree 5 poles (-14.970816, -0.935235) (-14.967309, -0.937482) (-14.960297, -0.941967) (-14.949781, -0.948677) (-14.935766, -0.957584) (-14.918257, -0.968655) (-14.900759, -0.979662) (-14.883271, -0.990605) (-14.865793, -1.001484) (-14.848325, -1.012299) (-14.830868, -1.02305) (-14.813423, -1.033738) (-14.795988, -1.044361) (-14.778565, -1.054921) (-14.761155, -1.065416) (-14.743756, -1.075848) (-14.72637, -1.086216) (-14.708998, -1.09652) (-14.691638, -1.10676) (-14.674292, -1.116936) (-14.65696, -1.127049) (-14.639642, -1.137097) (-14.622338, -1.147082) (-14.605049, -1.157003) (-14.587775, -1.166859) (-14.570516, -1.176652) (-14.553272, -1.186381) (-14.536045, -1.196047) (-14.518833, -1.205648) (-14.501638, -1.215186) (-14.48446, -1.22466) (-14.467299, -1.234069) (-14.450155, -1.243416) (-14.433029, -1.252698) (-14.415921, -1.261917) (-14.398832, -1.271072) (-14.381761, -1.280163) (-14.364708, -1.28919) (-14.347676, -1.298154) (-14.330662, -1.307054) (-14.313669, -1.315891) (-14.296696, -1.324663) (-14.279743, -1.333373) (-14.262812, -1.342018) (-14.245901, -1.3506) (-14.229012, -1.359119) (-14.212145, -1.367574) (-14.1953, -1.375965) (-14.178477, -1.384293) (-14.161678, -1.392558) (-14.144901, -1.400759) (-14.128148, -1.408897) (-14.111419, -1.416972) (-14.094714, -1.424983) (-14.078034, -1.432931) (-14.061379, -1.440816) (-14.044749, -1.448638) (-14.028144, -1.456396) (-14.011565, -1.464092) (-13.995013, -1.471724) (-13.978487, -1.479294) (-13.961988, -1.4868) (-13.945517, -1.494244) (-13.929073, -1.501624) (-13.912657, -1.508942) (-13.89627, -1.516197) (-13.879911, -1.523389) (-13.863582, -1.530519) (-13.847282, -1.537586) (-13.831012, -1.54459) (-13.814772, -1.551532) (-13.798563, -1.558412) (-13.782385, -1.565229) (-13.766238, -1.571984) (-13.750123, -1.578676) (-13.73404, -1.585306) (-13.71799, -1.591874) (-13.701972, -1.59838) (-13.685988, -1.604824) (-13.670038, -1.611206) (-13.654122, -1.617526) (-13.63824, -1.623785) (-13.622393, -1.629981) (-13.606581, -1.636116) (-13.590805, -1.64219) (-13.575065, -1.648201) (-13.559362, -1.654152) (-13.543695, -1.660041) (-13.528066, -1.665869) (-13.512475, -1.671635) (-13.496921, -1.677341) (-13.481407, -1.682985) (-13.465931, -1.688569) (-13.450495, -1.694092) (-13.435098, -1.699554) (-13.419742, -1.704955) (-13.404427, -1.710296) (-13.389152, -1.715577) (-13.37392, -1.720797) (-13.358729, -1.725956) (-13.343581, -1.731056) (-13.328475, -1.736096) (-13.313413, -1.741076) (-13.298395, -1.745996) (-13.283422, -1.750856) (-13.268493, -1.755657) (-13.253609, -1.760398) (-13.238771, -1.76508) (-13.223979, -1.769702) (-13.209233, -1.774266) (-13.194535, -1.77877) (-13.179884, -1.783216) (-13.165282, -1.787603) (-13.150728, -1.791932) (-13.136223, -1.796202) (-13.121768, -1.800413) (-13.107362, -1.804567) (-13.093007, -1.808662) (-13.078704, -1.8127) (-13.064451, -1.81668) (-13.050251, -1.820602) (-13.036104, -1.824467) (-13.02201, -1.828274) (-13.007969, -1.832025) (-12.993982, -1.835718) (-12.980051, -1.839355) (-12.966174, -1.842935) (-12.952353, -1.846458) (-12.938589, -1.849925) (-12.924882, -1.853337) (-12.911232, -1.856692) (-12.89764, -1.859991) (-12.884106, -1.863235) (-12.870632, -1.866424) (-12.857218, -1.869557) (-12.843864, -1.872635) (-12.830571, -1.875659) (-12.81734, -1.878627) (-12.80417, -1.881542) (-12.791064, -1.884402) (-12.77802, -1.887209) (-12.765041, -1.889961) (-12.752126, -1.89266) (-12.739277, -1.895306) (-12.726493, -1.897899) (-12.713776, -1.900438) (-12.701127, -1.902925) (-12.688544, -1.90536) (-12.676031, -1.907743) (-12.663586, -1.910074) (-12.651212, -1.912353) (-12.638908, -1.91458) (-12.626675, -1.916757) (-12.614514, -1.918883) (-12.602426, -1.920958) (-12.590411, -1.922983) (-12.57847, -1.924957) (-12.566604, -1.926883) (-12.554813, -1.928758) (-12.543099, -1.930585) (-12.531461, -1.932362) (-12.519902, -1.934091) (-12.508421, -1.935772) (-12.497019, -1.937405) (-12.485698, -1.938991) (-12.474458, -1.940529) (-12.463299, -1.94202) (-12.452223, -1.943465) (-12.44123, -1.944863) (-12.430322, -1.946216) (-12.419499, -1.947523) (-12.408762, -1.948785) (-12.398111, -1.950002) (-12.387549, -1.951175) (-12.377075, -1.952304) (-12.366691, -1.953389) (-12.356398, -1.954431) (-12.346195, -1.95543) (-12.336086, -1.956387) (-12.32607, -1.957303) (-12.316148, -1.958176) (-12.306322, -1.959009) (-12.296592, -1.959801) (-12.28696, -1.960554) (-12.277426, -1.961266) (-12.267992, -1.96194) (-12.258658, -1.962575) (-12.249427, -1.963171) (-12.240298, -1.963731) (-12.231273, -1.964253) (-12.222354, -1.964739) (-12.213541, -1.965189) (-12.204836, -1.965603) (-12.19624, -1.965983) (-12.187753, -1.966329) (-12.179378, -1.966641) (-12.171116, -1.96692) (-12.162968, -1.967167) (-12.154935, -1.967382) (-12.14702, -1.967567) (-12.139222, -1.967721) (-12.131544, -1.967845) (-12.123986, -1.967941) (-12.116552, -1.968009) (-12.109241, -1.968049) (-12.102057, -1.968063) (-12.094999, -1.968051) (-12.08807, -1.968014) (-12.081272, -1.967952) (-12.074606, -1.967868) (-12.068075, -1.967761) (-12.061679, -1.967633) (-12.05542, -1.967485) (-12.049302, -1.967316) (-12.043325, -1.96713) (-12.037491, -1.966925) (-12.031803, -1.966704) (-12.026262, -1.966468) (-12.020871, -1.966218) (-12.015633, -1.965954) (-12.010548, -1.965678) (-12.00562, -1.965392) (-12.000852, -1.965096) (-11.996245, -1.964792) (-11.991802, -1.964481) (-11.987526, -1.964165) (-11.983419, -1.963845) (-11.979485, -1.963522) (-11.975726, -1.963198) (-11.972145, -1.962875) (-11.968746, -1.962554) (-11.965532, -1.962238) (-11.962506, -1.961927) (-11.959673, -1.961624) (-11.957034, -1.961331) (-11.954593, -1.961049) (-11.952355, -1.96078) (-11.950325, -1.960527) (-11.948507, -1.960293) (-11.946908, -1.960081) (-11.945532, -1.959893) (-11.944609, -1.959763) (-11.944019, -1.959676) (-11.94367, -1.959624) (-11.943507, -1.959599) knots -1 -1 -1 -1 -1 -1 -0.99583333 -0.99166667 -0.9875 -0.98333333 -0.97916667 -0.975 -0.97083333 -0.96666667 -0.9625 -0.95833333 -0.95416667 -0.95 -0.94583333 -0.94166667 -0.9375 -0.93333333 -0.92916667 -0.925 -0.92083333 -0.91666667 -0.9125 -0.90833333 -0.90416667 -0.9 -0.89583333 -0.89166667 -0.8875 -0.88333333 -0.87916667 -0.875 -0.87083333 -0.86666667 -0.8625 -0.85833333 -0.85416667 -0.85 -0.84583333 -0.84166667 -0.8375 -0.83333333 -0.82916667 -0.825 -0.82083333 -0.81666667 -0.8125 -0.80833333 -0.80416667 -0.8 -0.79583333 -0.79166667 -0.7875 -0.78333333 -0.77916667 -0.775 -0.77083333 -0.76666667 -0.7625 -0.75833333 -0.75416667 -0.75 -0.74583333 -0.74166667 -0.7375 -0.73333333 -0.72916667 -0.725 -0.72083333 -0.71666667 -0.7125 -0.70833333 -0.70416667 -0.7 -0.69583333 -0.69166667 -0.6875 -0.68333333 -0.67916667 -0.675 -0.67083333 -0.66666667 -0.6625 -0.65833333 -0.65416667 -0.65 -0.64583333 -0.64166667 -0.6375 -0.63333333 -0.62916667 -0.625 -0.62083333 -0.61666667 -0.6125 -0.60833333 -0.60416667 -0.6 -0.59583333 -0.59166667 -0.5875 -0.58333333 -0.57916667 -0.575 -0.57083333 -0.56666667 -0.5625 -0.55833333 -0.55416667 -0.55 -0.54583333 -0.54166667 -0.5375 -0.53333333 -0.52916667 -0.525 -0.52083333 -0.51666667 -0.5125 -0.50833333 -0.50416667 -0.5 -0.49583333 -0.49166667 -0.4875 -0.48333333 -0.47916667 -0.475 -0.47083333 -0.46666667 -0.4625 -0.45833333 -0.45416667 -0.45 -0.44583333 -0.44166667 -0.4375 -0.43333333 -0.42916667 -0.425 -0.42083333 -0.41666667 -0.4125 -0.40833333 -0.40416667 -0.4 -0.39583333 -0.39166667 -0.3875 -0.38333333 -0.37916667 -0.375 -0.37083333 -0.36666667 -0.3625 -0.35833333 -0.35416667 -0.35 -0.34583333 -0.34166667 -0.3375 -0.33333333 -0.32916667 -0.325 -0.32083333 -0.31666667 -0.3125 -0.30833333 -0.30416667 -0.3 -0.29583333 -0.29166667 -0.2875 -0.28333333 -0.27916667 -0.275 -0.27083333 -0.26666667 -0.2625 -0.25833333 -0.25416667 -0.25 -0.24583333 -0.24166667 -0.2375 -0.23333333 -0.22916667 -0.225 -0.22083333 -0.21666667 -0.2125 -0.20833333 -0.20416667 -0.2 -0.19583333 -0.19166667 -0.1875 -0.18333333 -0.17916667 -0.175 -0.17083333 -0.16666667 -0.1625 -0.15833333 -0.15416667 -0.15 -0.14583333 -0.14166667 -0.1375 -0.13333333 -0.12916667 -0.125 -0.12083333 -0.11666667 -0.1125 -0.10833333 -0.10416667 -0.1 -0.09583333 -0.09166667 -0.0875 -0.08333333 -0.07916667 -0.075 -0.07083333 -0.06666667 -0.0625 -0.05833333 -0.05416667 -0.05 -0.04583333 -0.04166667 -0.0375 -0.03333333 -0.02916667 -0.025 -0.02083333 -0.01666667 -0.0125 -0.00833333 -0.00416667 0 0 0 0 0 0
  line L2 (-11.943507, -1.959599) -> (-11.942171, -1.959393)
  line L3 (-11.942171, -1.959393) -> (-9.251304, -1.517893)
  arc A2 (-9.251304, -1.517893) -> (-8.376657, -4.209779) centre (0, 0) ccw
  line L4 (-8.376657, -4.209779) -> (-10.813121, -5.43425)
  line L5 (-10.813121, -5.43425) -> (-10.814323, -5.434869)